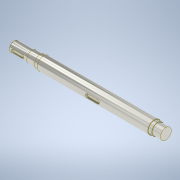
# Autodesk Inventor part: Валл
Saved by Autodesk Inventor 2021 (Build 250183000, 183)
## iProperties
Created: 2023-04-24
Part Number: Валл
Material: Сталь, углеродистая
Document SubType Name: Modeling
Designer: gdevc
Density: 7.85 g/cm^3
Appearance: Серебро
Author: gdevc
Autodesk Inventor part; units mm, degrees
ref_plane "YZ Plane" through (0, 0, 0) normal (1, 0, 0) x (0, 1, 0)
ref_plane "XZ Plane" through (0, 0, 0) normal (0, 1, 0) x (-1, 0, 0)
sketch "Эскиз1" plane through (0, 0, 0) normal (0, 0, 1) x (1, 0, 0)
  line L0 (0, 0) -> (761, 0)
  line L1 (0, 0) -> (0, 25)
  line L2 (0, 25) -> (90, 25)
  line L3 (90, 25) -> (90, 27.5)
  line L4 (90, 27.5) -> (131, 27.5)
  line L5 (131, 27.5) -> (131, 30)
  line L6 (425.5, 30) -> (425.5, 0) construction
  line L7 (720, 27.5) -> (720, 30)
  line L8 (131, 30) -> (148, 30)
  line L9 (148, 30) -> (148, 32.5)
  line L10 (148, 32.5) -> (181, 32.5)
  line L11 (720, 30) -> (703, 30)
  line L12 (703, 30) -> (703, 32.5)
  line L13 (703, 32.5) -> (181, 32.5)
  line L14 (720, 27.5) -> (761, 27.5)
  line L15 (761, 27.5) -> (761, 0)
  dimension "d0" = 50
  dimension "d1" = 55
  dimension "d2" = 90
  dimension "d3" = 41
  dimension "d14" = 17
  dimension "d15" = 60
  dimension "d16" = 65
  dimension "d27" = 41
  dimension "d29" = 630
  constraints: 32 end point, 5 vertical, 4 perpendicular, 4 symmetric about line, 3 horizontal
  measures "d0" diameter of L2 L0
  measures "d1" diameter of L4 L0
  measures "d2" distance from line of L0.start L3
  measures "d3" distance of L3.end L4.end
  measures "d14" distance of L5.end L8.end
  measures "d15" diameter of L8 L0
  measures "d16" diameter of L10 L0
  measures "d27" distance of L7.start L14.end
  measures "d29" distance between parallel lines of L7 L3
revolve "Вращение1" add sketch "Эскиз1" angle 360 about axis through (0, 0, 0) along (1, 0, 0)
ref_plane "РабПлоскость1" through (0, 0, 19) normal (0, 0, 1) x (1, 0, 0)
sketch "Эскиз2" plane through (0, 0, 19) normal (0, 0, 1) x (1, 0, 0)
  line L0 (65, 8) -> (20, 8)
  line L1 (20, 8) -> (20, -8)
  line L2 (20, -8) -> (65, -8)
  line L3 (65, -8) -> (65, 8)
  arc A0 (65, -8) -> (65, 8) centre (65, 0) ccw
  arc A1 (20, 8) -> (20, -8) centre (20, 0) ccw
  point P0 (0, 0)
  dimension "d8" = 8
  dimension "d9" = 16
  dimension "d10" = 45
  dimension "d11" = 20
  constraints: 8 end point, 4 point on circle, 2 centre point, 2 midpoint, 2 parallel, 1 horizontal, 1 perpendicular
  measures "d8" distance from line of point (0, 0) L0
  measures "d9" distance between parallel lines of L2 L0
  measures "d10" distance between parallel lines of L1 L3
  measures "d11" distance from line of point (0, 0) L1
extrude "Выдавливание1" cut sketch "Эскиз2" along normal blind 33
ref_plane "РабПлоскость2" through (0, 0, 25.5) normal (0, 0, 1) x (1, 0, 0)
sketch "Эскиз3" plane through (0, 0, 25.5) normal (0, 0, 1) x (1, 0, 0)
  line L0 (148, -32.5) -> (148, 32.5) projected
  line L1 (400.5, 9) -> (450.5, 9)
  line L2 (450.5, 9) -> (450.5, -9)
  line L3 (450.5, -9) -> (400.5, -9)
  line L4 (400.5, -9) -> (400.5, 9)
  arc A0 (400.5, 9) -> (400.5, -9) centre (400.5, 0) ccw
  arc A1 (450.5, -9) -> (450.5, 9) centre (450.5, 0) ccw
  line L5 (703, -30) -> (703, 30) projected
  point P0 (0, 0)
  dimension "d19" = 18
  dimension "d20" = 252.5
  dimension "d21" = 50
  dimension "d22" = 9
  dimension "d26" = 555
  constraints: 8 end point, 4 point on circle, 2 centre point, 2 midpoint, 2 parallel, 1 horizontal, 1 perpendicular
  measures "d19" distance between parallel lines of L3 L1
  measures "d20" distance between parallel lines of L0 L4
  measures "d21" distance between parallel lines of L2 L4
  measures "d22" vertical distance of point (0, 0) L3.end
  measures "d26" distance between parallel lines of L5 L0
extrude "Выдавливание2" cut sketch "Эскиз3" along normal blind 44.75
chamfer "Фаска1" distance 2 angle 45 1 edges at (0, -25, 0)
equation "\"d27\" = d3"
equation "\"d8\" = 0.5 * d9"
equation "\"d22\" = 0.5 * d19"
